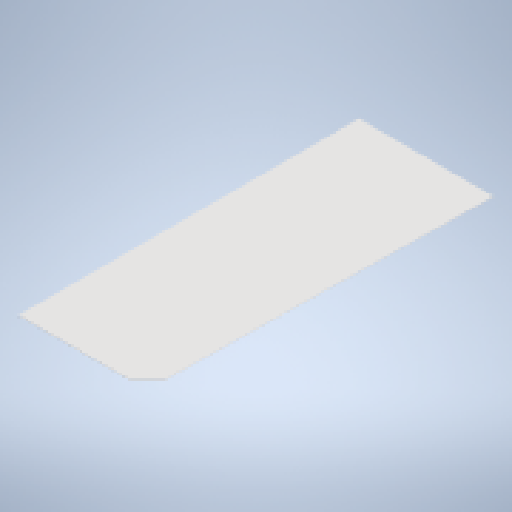
# Autodesk Inventor part: BSH 039 back 9
Saved by Autodesk Inventor 2025 (Build 290162010, 162A)
## iProperties
Created: 2024-07-23
Part Number: BSH 039 back 9
Material: Water
Document SubType Name: Sheet Metal
Designer: admin
Mass: 2.72236e+06 g
Surface Area: 129470 cm^2
Volume: 2.727e+06 cm^3
Density: 0.9983 g/cm^3
Sheet Metal Rule: AISI304 3mm Die 32
Sheet Metal Width: 0,000 mm
Sheet Metal Length: 0,000 mm
Sheet Metal Area: 0,000 mm^2
Appearance: Default
Author: admin
Autodesk Inventor part; units mm, degrees
ref_plane "YZ Plane" through (0, 0, 0) normal (1, 0, 0) x (0, 1, 0)
ref_plane "XZ Plane" through (0, 0, 0) normal (0, 1, 0) x (-1, 0, 0)
ref_plane "XY Plane" through (0, 0, 0) normal (0, 0, 1) x (1, 0, 0)
sketch "Sketch5" plane through (0, 0, 0) normal (0, 0, 1) x (1, 0, 0)
  line L0 (0, 2900) -> (1200, 2900)
  line L1 (1200, 2900) -> (1200, 0)
  line L2 (1200, 0) -> (0, 0)
  line L3 (0, 0) -> (0, 2900)
  line L4 (0, 2900) -> (1200, 0) construction
  line L5 (1200, 2900) -> (0, 0) construction
  line L6 (950, 0) -> (1100, 150)
  line L7 (1100, 150) -> (1147, 2900)
  line L8 (-1308.8025, 1126.8027) -> (-1508.8025, 1126.8027)
  line L9 (-1508.8025, 1126.8027) -> (-2408.8025, 2126.8027)
  line L10 (-2408.8025, 2126.8027) -> (-2408.8025, 4026.8027)
  line L11 (-2408.8025, 4026.8027) -> (-1108.8025, 4026.8027)
  line L12 (-1108.8025, 4026.8027) -> (-1308.8025, 1126.8027)
  point P0 (600, 1450)
  dimension "d26" = 1200
  dimension "d27" = 2900
  dimension "d29" = 53
  dimension "d30" = 950
  dimension "d31" = 150
  dimension "d32" = 100
  dimension "d33" = 200
  dimension "d34" = 1000
  dimension "d35" = 1300
  dimension "d36" = 1900
  dimension "d37" = 900
  constraints: 26 end point, 3 perpendicular, 2 horizontal, 2 midpoint, 2 parallel, 2 point on line, 1 coincident
  measures "d26" distance of L1.end L2.end
  measures "d27" distance of L0.end L1.end
  measures "d29" distance of L0.end L7.end
  measures "d30" distance of point (0, 0) L6.start
  measures "d31" distance from line of L2 L6.end
  measures "d32" distance from line of L1 L6.end
  measures "d33" distance of L8.start L8.end
  measures "d34" distance from line of L9.end L8
  measures "d35" distance of L11.end L10.end
  measures "d36" distance of L9.end L10.end
  measures "d37" horizontal distance of L8.end L9.end
extrude "Extrusion2" add sketch "Sketch5" along normal blind 900 contours L8 L9 L10 L11 L12
equation "\"BendReliefWidth\" = Thickness"
equation "\"BendReliefDepth\" = 0.5 * Thickness"
equation "\"CornerReliefSize\" = 4 * Thickness"
equation "\"MinimumRemnant\" = 2 * Thickness"
equation "\"TransitionRadius\" = BendRadius"
equation "\"JacobiRadiusSize\" = BendRadius"
equation "\"GapSize\" = Thickness"
equation "\"Thickness\" = 3"
equation "\"BendRadius\" = 5"
body "Solid3"
